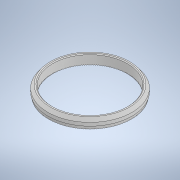
# Autodesk Inventor part: Retaining ring
Saved by Autodesk Inventor 2020.5 (Build 245400000, 400)
## iProperties
Created: 2024-03-01
Part Number: Retaining ring
Material: Generic
Document SubType Name: Modeling
Designer: aivel
Density: 1 g/cm^3
Appearance: Default
Author: aivel
Autodesk Inventor part; units mm, degrees
ref_plane "YZ Plane" through (0, 0, 0) normal (1, 0, 0) x (0, 1, 0)
ref_plane "XZ Plane" through (0, 0, 0) normal (0, 1, 0) x (-1, 0, 0)
ref_plane "XY Plane" through (0, 0, 0) normal (0, 0, 1) x (1, 0, 0)
sketch "Sketch1" plane through (0, 0, 0) normal (0, 1, 0) x (-1, 0, 0)
  circle A0 centre (0, 0) radius 11.35
  circle A1 centre (0, 0) radius 12.75
  dimension "d0" = 22.7
  dimension "d1" = 25.5
  constraints: 2 centre point, 2 coincident
  measures "d0" diameter of A0
  measures "d1" diameter of A1
extrude "Extrusion1" add sketch "Sketch1" along normal blind 3
chamfer "Chamfer1" distance 0.25 angle 45 1 edges at (11.35, 3, 0)
chamfer "Chamfer2" distance 1 distance2 0.25 1 edges at (12.75, 0, 0) measured on face at (-12.7087, 2, -1.0259)
chamfer "Chamfer3" distance 0.75 distance2 1 1 edges at (12.75, 3, 0) measured on face at (-12.1308, 3, -1.9424)
sketch "Sketch5" plane through (0, 0, 0) normal (0, -1, 0) x (1, 0, 0)
  line L0 (0, 0) -> (-0.2243, -12.848)
  line L1 (0, 0) -> (0.2243, -12.848)
  arc A0 (-0.2243, -12.848) -> (0.2243, -12.848) centre (0, 0) ccw
  constraints: 4 end point, 2 point on circle, 1 centre point, 1 coincident
extrude "Extrusion3" cut sketch "Sketch5" against normal blind 0.2 draft -45
pattern_circular "Circular Pattern2" count 180 over 360 about axis through (0, 0, 0) along (0, 1, 0) of "Extrusion3"
body "Solid1"
